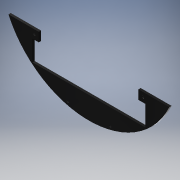
# Autodesk Inventor part: va
Saved by Autodesk Inventor 2017 (Build 210142000, 142)
## iProperties
Part Number: va
Material: Genérico
Document SubType Name: Modeling
Designer: Roberto
Density: 1 g/cm^3
Appearance: Valor por defecto
Author: Roberto
Autodesk Inventor part; units mm, degrees
ref_plane "Plano de trabajo1" through (-3.6477, -5.1016, -7.3334) normal (0, 1, 0) x (1, 0, 0)
sketch "Boceto1" plane through (-3.6477, -5.1016, -7.3334) normal (0, 1, 0) x (1, 0, 0)
  line L0 (5.2883, -3.4507) -> (5.2882, -3.8566) projected
  line L1 (4.7883, -3.4507) -> (5.2883, -3.4507) projected
  line L2 (5.2882, -3.8566) -> (5.2882, -4.1566) projected
  line L3 (5.2881, -4.2507) -> (4.0881, -4.2506) projected
  line L4 (-3.5114, -3.8566) -> (-3.5113, -4.1566) projected
  line L5 (-3.5114, -3.8566) -> (-3.5116, -3.451) projected
  line L6 (-3.5116, -3.451) -> (-3.0116, -3.4508) projected
  line L7 (-3.7131, -1.2144) -> (-2.2169, -0.3506) projected
  line L8 (-6.2177, -4.3514) -> (-5.3539, -2.8553) projected
  line L9 (7.1305, -2.8553) -> (7.9943, -4.3514) projected
  line L10 (3.9936, -0.3506) -> (5.4897, -1.2144) projected
  line L11 (0.0245, 0.25) -> (1.7521, 0.25) projected
  arc A0 (7.9495, -4.2507) -> (-6.173, -4.251) centre (0.8883, -7.4566) ccw
  line L12 (-2.3112, -4.2505) -> (-3.5112, -4.251) projected
  line L13 (5.2881, -4.2507) -> (7.9495, -4.2507)
  line L14 (-3.5112, -4.251) -> (-6.173, -4.251)
  line L15 (-3.5112, -4.251) -> (-3.5116, -3.451)
  line L16 (-3.5116, -3.451) -> (5.2883, -3.4507)
  line L17 (5.2883, -3.4507) -> (5.2881, -4.2507)
  point P0 (3.6477, -7.3334)
  constraints: 10 end point, 3 point on circle, 2 horizontal, 1 centre point
extrude "Extrusión1" add sketch "Boceto1" along normal blind 0.2
ref_plane "Plano de trabajo2" through (-3.6477, -4.9016, -7.3334) normal (0, 1, 0) x (1, 0, 0)
sketch "Boceto2" plane through (-3.6477, -4.9016, -7.3334) normal (0, 1, 0) x (1, 0, 0)
  line L0 (5.0906, -1.7512) -> (-3.3106, -1.7469) projected
  line L1 (-3.3106, -1.8516) -> (-3.9207, -1.8515) projected
  line L2 (5.8384, -2.2498) -> (5.8385, -2.023) projected
  line L3 (-4.0622, -2.0234) -> (-4.0621, -2.2502) projected
  line L4 (5.8385, -2.023) -> (5.8385, -4.7089)
  line L5 (-4.0622, -2.0234) -> (-4.0622, -5.784)
  line L6 (5.0906, -1.7512) -> (-3.3106, -1.7469)
  line L7 (5.8385, -2.023) -> (5.8385, -1.7512)
  line L8 (5.8385, -1.7512) -> (5.0906, -1.7512)
  line L9 (-3.3106, -1.7469) -> (-4.0637, -1.7512)
  line L10 (-4.0637, -1.7512) -> (-4.0622, -2.0234)
  line L11 (5.8385, -4.7089) -> (-4.0637, -4.7089)
  line L12 (-4.0637, -4.7089) -> (-4.0637, -1.7512)
  line L13 (-4.0637, -1.7512) -> (5.8385, -1.7512)
  line L14 (5.8385, -1.7512) -> (5.8385, -4.7089)
  line L15 (5.0906, -1.6539) -> (-3.3105, -1.6519) projected
  line L16 (-4.0637, -1.7512) -> (5.8385, -1.7512)
  line L17 (5.8385, -1.7512) -> (5.8385, -1.654)
  line L18 (5.8385, -1.654) -> (-4.0637, -1.654)
  line L19 (-4.0637, -1.654) -> (-4.0637, -1.7512)
  point P0 (3.6477, -7.3334)
  point P1 (-3.2616, -3.4509)
  constraints: 30 end point, 4 parallel, 4 perpendicular, 3 vertical, 2 horizontal, 1 point on line
extrude "Extrusión2" cut sketch "Boceto2" against normal blind 0.2
ref_plane "Plano de trabajo3" through (-7.1593, -4.0366, -3.8824) normal (-1, 0, 0.0004) x (0.0004, 0, 1)
sketch "Boceto3" plane through (-7.1593, -4.0366, -3.8824) normal (-1, 0, 0.0004) x (0.0004, 0, 1)
  line L0 (0.7998, -1.065) -> (0.7998, -0.865) projected
  line L1 (-1.7972, -1.065) -> (0.7998, -1.065) projected
  line L2 (-1.7972, -0.865) -> (-1.7972, -1.065) projected
  line L3 (0.7998, -0.865) -> (-1.7972, -0.865) projected
  line L4 (0, -1.065) -> (0, -0.4397)
  line L5 (0.7998, -0.865) -> (0, -0.865)
  line L6 (0, -0.865) -> (0, -1.065)
  line L7 (0, -1.065) -> (0.7998, -1.065)
  line L8 (0.7998, -1.065) -> (0.7998, -0.865)
  point P0 (3.8854, 4.0366)
  constraints: 10 end point, 2 parallel, 2 perpendicular, 1 horizontal
extrude "Extrusión3" add sketch "Boceto3" along normal blind 0.6 contours L1 L4 L3 L0
ref_plane "Plano de trabajo4" through (2.1908, -4.9016, -5.3103) normal (-1, 0, 0) x (0, 0, 1)
sketch "Boceto4" plane through (2.1908, -4.9016, -5.3103) normal (-1, 0, 0) x (0, 0, 1)
  line L0 (2.2277, -0.2) -> (2.2277, 0) projected
  line L1 (1.4279, 0) -> (1.4279, -0.2) projected
  line L2 (2.2277, 0) -> (1.4279, 0) projected
  line L3 (1.4279, -0.2) -> (2.2277, -0.2) projected
  point P0 (5.3103, 4.9016)
extrude "Extrusión4" add sketch "Boceto4" along normal blind 0.6
sketch "Boceto5" plane through (-3.6477, -4.9016, -7.3334) normal (0, 1, 0) x (1, 0, 0)
  line L0 (-3.5116, -3.451) -> (-3.5112, -4.2507) projected
  line L1 (-3.5112, -4.2507) -> (-4.3112, -4.251)
  line L2 (-4.1112, -4.251) -> (-6.173, -4.251) projected
  line L3 (-3.5116, -3.451) -> (-3.5112, -4.2507)
  circle A0 centre (-3.9114, -3.851) radius 0.1
  line L4 (5.2385, -3.451) -> (5.2385, -4.2507) projected
  line L5 (5.2385, -3.451) -> (5.2385, -4.2507)
  line L6 (5.2385, -4.2507) -> (6.0385, -4.2507)
  line L7 (5.8385, -4.2507) -> (7.9495, -4.2507) projected
  line L8 (5.8385, -3.451) -> (5.2385, -3.451) projected
  circle A1 centre (5.6385, -3.8509) radius 0.1
  point P0 (3.6477, -7.3334)
  dimension "d9" = 0.8
  dimension "d10" = 0.2
  dimension "d11" = 0.8
  dimension "d12" = 0.2
  constraints: 8 end point, 2 centre point, 2 point on line, 1 vertical
  measures "d9" distance of L0.end L1.end
  measures "d10" diameter of A0
  measures "d11" distance of L4.end L6.end
  measures "d12" diameter of A1
extrude "Extrusión5" cut sketch "Boceto5" against normal blind 0.6
sketch "Boceto6" plane through (-3.6477, -5.1016, -7.3334) normal (0, -1, 0) x (1, 0, 0)
  circle A0 centre (-0.9872, 0.207) radius 0.1 projected
  circle A1 centre (2.7638, 0.207) radius 0.1 projected
  point P0 (3.6477, 7.3334)
extrude "Extrusión6" cut sketch "Boceto6" against normal blind 1
